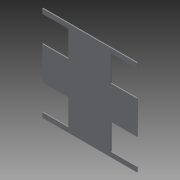
# Autodesk Inventor part: Bodenplatte
Saved by Autodesk Inventor 2014 (Build 180170000, 170)
## iProperties
Created: 2015-11-27
Part Number: Bodenplatte
Material: Generisch
Document SubType Name: Modeling
Designer: nrk
Density: 1 g/cm^3
Appearance: Vorgabe
Author: nrk
Autodesk Inventor part; units mm, degrees
ref_plane "YZ Plane" through (0, 0, 0) normal (1, 0, 0) x (0, 1, 0)
ref_plane "XZ Plane" through (0, 0, 0) normal (0, 1, 0) x (-1, 0, 0)
ref_plane "XY Plane" through (0, 0, 0) normal (0, 0, 1) x (1, 0, 0)
sketch "Skizze1" plane through (0, 0, 0) normal (0, 1, 0) x (-1, 0, 0)
  line L0 (-90, 200) -> (90, 200)
  line L1 (90, -200) -> (-90, -200)
  line L2 (-90, 200) -> (90, -200) construction
  line L3 (90, 200) -> (-90, -200) construction
  line L4 (-90, 200) -> (-200, 200)
  line L5 (-200, 200) -> (-200, 180)
  line L6 (-200, 180) -> (-90, 180)
  line L7 (90, 200) -> (200, 200)
  line L8 (200, 200) -> (200, 180)
  line L9 (200, 180) -> (90, 180)
  line L10 (-90, -200) -> (-200, -200)
  line L11 (-200, -200) -> (-200, -180)
  line L12 (-200, -180) -> (-90, -180)
  line L13 (90, -200) -> (200, -200)
  line L14 (200, -200) -> (200, -180)
  line L15 (200, -180) -> (90, -180)
  line L16 (-90, -70) -> (-200, -70)
  line L17 (-200, -70) -> (-200, 70)
  line L18 (-200, 70) -> (-90, 70)
  line L19 (233.2705, 0) -> (-241.4406, 0)
  line L20 (0, 254.3005) -> (0, -301.4948)
  line L21 (90, 70) -> (200, 70)
  line L22 (200, 70) -> (200, -70)
  line L23 (200, -70) -> (90, -70)
  line L24 (-90, -180) -> (-90, -70)
  line L25 (-90, 70) -> (-90, 180)
  line L26 (90, 180) -> (90, 70)
  line L27 (90, -70) -> (90, -180)
  point P0 (0, 0)
  point P1 (-90, 0)
  dimension "d17" = 180
  dimension "d19" = 110
  dimension "d20" = 110
  dimension "d23" = 140
  dimension "d25" = 20
  constraints: 56 end point, 9 parallel, 9 perpendicular, 6 horizontal, 5 collinear, 2 midpoint, 5 other
  measures "d17" distance of L1.start L1.end
  measures "d19" distance of L6.end L5.end
  measures "d20" distance of L9.end L8.end
  measures "d23" distance of L16.start L18.end
  measures "d25" distance of L5.end L4.end
extrude "Extrusion1" add sketch "Skizze1" along normal blind 4
